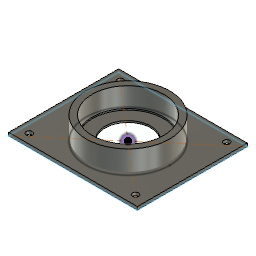
bearing holder ground (Autodesk Fusion 360 design; units mm, degrees)
part number: 2026-01-16-12-08-01-742
Autodesk Fusion 360 part; units mm, degrees
sketch "Sketch1" plane through (0, 0, 0) normal (0, 0, 1) x (1, 0, 0)
  circle A0 centre (0, 0) radius 27.5
  line L0 (42.3621, 36.2343) -> (-42.3621, 36.2343)
  line L1 (-42.3621, 36.2343) -> (-42.3621, -36.2343)
  line L2 (-42.3621, -36.2343) -> (42.3621, -36.2343)
  line L3 (42.3621, -36.2343) -> (42.3621, 36.2343)
  line L4 (42.3621, 36.2343) -> (-42.3621, -36.2343) construction
  line L5 (-42.3621, 36.2343) -> (42.3621, -36.2343) construction
  dimension "d1" = 55
  constraint coincident A0.centre origin
  constraint horizontal L0
  constraint perpendicular L0 L1
  constraint parallel L0 L2
  constraint parallel L1 L3
  constraint coincident L4 A0.centre
  constraint coincident L5 A0.centre
  measures "d1" diameter of A0
extrude "Extrude1" add sketch "Sketch1" along normal blind 2 contours A0 | L0 L1 L2 L3 makes body 1
extrude "Extrude2" add sketch "Sketch1" along normal blind 15 separate body contours A0 makes body 2
sketch "Sketch2" plane through (0, 0, 15) normal (0, 0, 1) x (-1, 0, 0)
  circle A0 centre (0, 0) radius 27.5
  circle A1 centre (0, 0) radius 23.5
  dimension "d6" = 47
  constraint coincident A0.centre A1.centre
  measures "d6" diameter of A1
extrude "Extrude3" cut sketch "Sketch2" against normal blind 13.9 contours A1 bodies 1 2
sketch "Sketch3" plane through (0, 0, 2) normal (0, 0, 1) x (-1, 0, 0)
  circle A0 centre (0, 0) radius 23.5
  line L0 (-42.3621, 36.2343) -> (-42.3621, -36.2343)
  line L1 (-42.3621, -36.2343) -> (42.3621, -36.2343)
  line L2 (42.3621, -36.2343) -> (42.3621, 36.2343)
  line L3 (42.3621, 36.2343) -> (-42.3621, 36.2343)
  circle A1 centre (35, -30) radius 2
  circle A2 centre (-35, -30) radius 2
  circle A3 centre (35, 30) radius 2
  circle A4 centre (-35, 30) radius 2
  dimension "d9" = 4
  dimension "d10" = 4
  dimension "d11" = 4
  dimension "d12" = 4
  measures "d9" diameter of A1
  measures "d10" diameter of A2
  measures "d11" diameter of A3
  measures "d12" diameter of A4
extrude "Extrude4" cut sketch "Sketch3" against normal blind 2 contours A1 | A2 | A3 | A4 bodies 1
sketch "Sketch4" plane through (0, 0, 0) normal (0, 0, 1) x (1, 0, 0)
  circle A0 centre (0, 0) radius 15
  dimension "d15" = 30
  constraint coincident A0.centre origin
  measures "d15" diameter of A0
extrude "Extrude5" cut sketch "Sketch4" along normal blind 12 bodies 1 2
